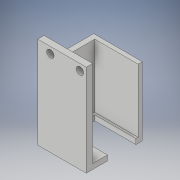
# Autodesk Inventor part: SOPORTE_HOTEND
Saved by Autodesk Inventor 2019 (Build 230136000, 136)
## iProperties
Created: 2020-09-19
Part Number: SOPORTE_HOTEND
Material: Generic
Document SubType Name: Modeling
Designer: ASUS
Density: 1 g/cm^3
Appearance: Default
Author: ASUS
Autodesk Inventor part; units mm, degrees
ref_plane "YZ Plane" through (0, 0, 0) normal (1, 0, 0) x (0, 1, 0)
ref_plane "XZ Plane" through (0, 0, 0) normal (0, 1, 0) x (-1, 0, 0)
ref_plane "XY Plane" through (0, 0, 0) normal (0, 0, 1) x (1, 0, 0)
sketch "Sketch1" plane through (0, 0, 0) normal (0, 0, 1) x (1, 0, 0)
  line L0 (0, 0) -> (23, 0)
  line L1 (23, 0) -> (23, 43.5)
  line L2 (23, 43.5) -> (0, 43.5)
  line L3 (0, 43.5) -> (0, 0)
  dimension "d0" = 23
  dimension "d1" = 43.5
  constraints: 8 end point, 2 parallel, 1 horizontal, 1 perpendicular
  measures "d0" distance of L2.end L1.end
  measures "d1" distance of L1.end L0.end
extrude "Extrusion1" add sketch "Sketch1" along normal blind 3
sketch "Sketch6" plane through (0, 0, 0) normal (0, 0, -1) x (-1, 0, 0)
  line L0 (0, 0) -> (-2.5, 0)
  line L1 (-2.5, 0) -> (-2.5, 32.5)
  line L2 (-2.5, 32.5) -> (0, 32.5)
  line L3 (0, 32.5) -> (0, 0)
  dimension "d17" = 2.5
  dimension "d18" = 32.5
  constraints: 8 end point, 2 parallel, 1 horizontal, 1 perpendicular
  measures "d17" distance of L1.end L2.end
  measures "d18" distance of L0.end L1.end
extrude "Extrusion5" add sketch "Sketch6" along normal blind 23.5
sketch "Sketch7" plane through (2.5, 0, 0) normal (1, 0, 0) x (0, 0, -1)
  line L0 (23.5, 0) -> (23.5, 32.5) projected
  line L1 (0, 32.5) -> (23.5, 32.5) projected
  line L2 (23.5, 0) -> (21.5, 0)
  line L3 (21.5, 0) -> (21.5, 32.5)
  line L4 (21.5, 32.5) -> (23.5, 32.5)
  line L5 (23.5, 32.5) -> (23.5, 0)
  point P0 (0, 0)
  dimension "d21" = 2
  constraints: 8 end point, 2 parallel, 1 horizontal, 1 perpendicular, 1 point on line
  measures "d21" distance of L3.end L4.end
extrude "Extrusion6" add sketch "Sketch7" along normal blind 20.5
sketch "Sketch8" plane through (0, 0, 3) normal (0, -1, 0) x (1, 0, 0)
  line L0 (2.5, -3) -> (23, -3) projected
  line L1 (23, -3) -> (23, 0) projected
  line L2 (0, 0) -> (23, 0) projected
  line L3 (0, 0) -> (0, -26.5) projected
  line L4 (0, -26.5) -> (23, -26.5) projected
  line L5 (23, -24.5) -> (23, -26.5) projected
  line L6 (2.5, -24.5) -> (23, -24.5) projected
  line L7 (2.5, -3) -> (2.5, -24.5) projected
  line L8 (23, -3) -> (23, -10)
  line L9 (23, -10) -> (7.5, -10)
  line L10 (7.5, -10) -> (7.5, -23.5)
  line L11 (7.5, -23.5) -> (23, -23.5)
  line L12 (23, -23.5) -> (23, -24.5)
  point P0 (0, -3)
  dimension "d24" = 7
  dimension "d25" = 1
  dimension "d26" = 5
  constraints: 10 end point, 4 perpendicular, 1 point on line, 1 vertical
  measures "d24" distance between parallel lines of L0 L9
  measures "d25" distance between parallel lines of L6 L11
  measures "d26" distance between parallel lines of L7 L10
extrude "Extrusion7" add sketch "Sketch8" against normal blind 2.5 contours L0 L8 L9 L10 L11 L12 L6 L7
sketch "Sketch10" plane through (0, 2.5, 3) normal (0, 1, 0) x (1, 0, 0)
  circle A0 centre (13, 7.5) radius 2
  line L0 (23, 3) -> (23, 10) projected
  line L1 (23, 3) -> (0, 3) projected
  dimension "d35" = 10
  dimension "d36" = 4.5
  dimension "d37" = 4
  constraints: 1 centre point
  measures "d35" distance from line of L0 A0.centre
  measures "d36" distance from line of L1 A0.centre
  measures "d37" diameter of A0
extrude "Extrusion9" cut sketch "Sketch10" against normal blind 2.5
sketch "Sketch11" plane through (0, 0, 3) normal (0, 0, 1) x (1, 0, 0)
  circle A0 centre (6, 40.5) radius 1.75
  circle A1 centre (20, 40.5) radius 1.75
  line L0 (0, 43.5) -> (0, 0) projected
  line L1 (23, 0) -> (23, 43.5) projected
  line L2 (0, 0) -> (23, 0) projected
  dimension "d40" = 3.5
  dimension "d41" = 3.5
  dimension "d42" = 14
  dimension "d44" = 3
  dimension "d45" = 40.5
  constraints: 2 centre point, 1 horizontal alignment
  measures "d40" diameter of A0
  measures "d41" diameter of A1
  measures "d42" distance of A1.centre A0.centre
  measures "d44" distance from line of L1 A1.centre
  measures "d45" distance from line of L2 A1.centre
extrude "Extrusion10" cut sketch "Sketch11" against normal blind 3
sketch "Sketch12" plane through (0, 0, 3) normal (0, -1, 0) x (1, 0, 0)
  line L0 (23, -23.5) -> (7.5, -23.5) projected
  line L1 (7.5, -23.5) -> (3.5, -23.5)
  line L2 (3.5, -23.5) -> (3.5, -17.5)
  line L3 (3.5, -17.5) -> (7.5, -17.5)
  line L4 (7.5, -17.5) -> (7.5, -23.5)
  point P0 (0, -3)
  dimension "d48" = 4
  dimension "d49" = 6
  constraints: 8 end point, 2 parallel, 1 horizontal, 1 perpendicular
  measures "d48" distance of L2.end L3.end
  measures "d49" distance of L1.end L2.end
extrude "Extrusion11" cut sketch "Sketch12" against normal blind 2.5
equation "\"d41\" = d40"
body "Solid1"
